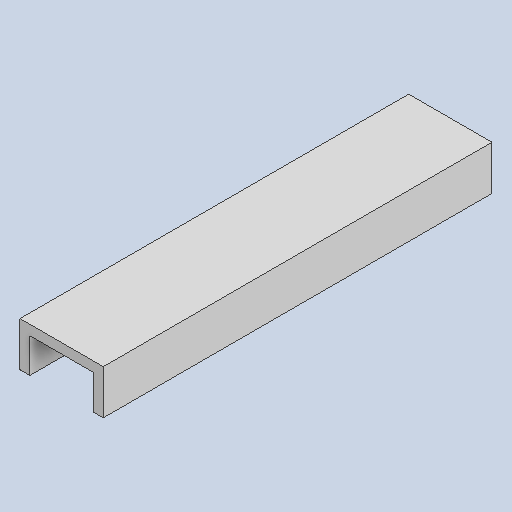
# Autodesk Inventor part: LongC3x6Top14in
Saved by Autodesk Inventor 2023 (Build 270158030, 158C)
## iProperties
Created: 2022-06-29
Part Number: LongC3x6Top14in
Material: Generic
Document SubType Name: Modeling
Designer: jeremyy
Density: 1 g/cm^3
Appearance: Default
Author: jeremyy
Autodesk Inventor part; units mm, degrees
ref_plane "YZ Plane" through (0, 0, 0) normal (1, 0, 0) x (0, 1, 0)
ref_plane "XZ Plane" through (0, 0, 0) normal (0, 1, 0) x (-1, 0, 0)
ref_plane "XY Plane" through (0, 0, 0) normal (0, 0, 1) x (1, 0, 0)
sketch "Sketch1" plane through (0, 0, 0) normal (0, 0, 1) x (1, 0, 0)
  line L0 (0, 0) -> (76.2, 0)
  line L1 (76.2, 0) -> (76.2, -40.5384)
  line L2 (76.2, -40.5384) -> (67.1576, -40.5384)
  line L3 (67.1576, -40.5384) -> (67.1576, -9.0424)
  line L4 (67.1576, -9.0424) -> (9.0424, -9.0424)
  line L5 (9.0424, -9.0424) -> (9.0424, -40.5384)
  line L6 (9.0424, -40.5384) -> (0, -40.5384)
  line L7 (0, -40.5384) -> (0, 0)
  dimension "d0" = 76.2
  dimension "d1" = 40.5384
  dimension "d2" = 9.0424
  dimension "d3" = 9.0424
  dimension "d4" = 9.0424
  constraints: 16 end point, 6 perpendicular, 2 point on line, 1 horizontal
  measures "d0" distance of L0.start L0.end
  measures "d1" distance of L0.end L1.end
  measures "d2" distance of L1.end L2.end
  measures "d3" distance of L5.end L6.end
  measures "d4" distance between parallel lines of L0 L4
extrude "Extrusion1" add sketch "Sketch1" along normal blind 355.6
body "Solid1"
